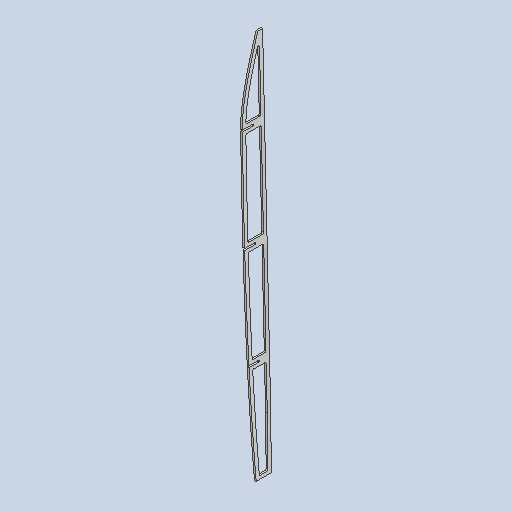
# Autodesk Inventor part: stringer_cowl
Saved by Autodesk Inventor 2022 (Build 260153000, 153)
## iProperties
Created: 2021-05-01
Part Number: stringer_cowl
Material: Generic
Document SubType Name: Modeling
Designer: kardo
Density: 1 g/cm^3
Appearance: Default
Mass: 8.25745 g
Surface Area: 121.112 cm^2
Volume: 8.25745 cm^3
Author: kardo
Autodesk Inventor part; units mm, degrees
ref_plane "YZ Plane" through (0, 0, 0) normal (1, 0, 0) x (0, 1, 0)
ref_plane "XZ Plane" through (0, 0, 0) normal (0, 1, 0) x (-1, 0, 0)
ref_plane "XY Plane" through (0, 0, 0) normal (0, 0, 1) x (1, 0, 0)
derived "frame_outline.ipt"
sketch "stringer_cowl" plane through (55, 0, 0) normal (1, 0, 0) x (0, 1, 0)
  line L0 (-363, 18.496) -> (-297.6664, 19.4083)
  line L1 (-37.9005, 25.6108) -> (-277.6703, 19.7906)
  line L2 (28.4595, 27.2216) -> (-37.9005, 25.6108)
  line L3 (94.8, 28.832) -> (28.4595, 27.2216)
  line L4 (-361, 19.324) -> (-297.6775, 20.2082)
  line L5 (-277.6897, 20.5903) -> (-37.9199, 26.4106)
  line L6 (-37.9199, 26.4106) -> (28.4401, 28.0214)
  line L7 (28.4401, 28.0214) -> (92.8, 29.5837)
  line L8 (-361, 19.324) -> (-361, 37.0229)
  line L9 (92.8, 35.2245) -> (92.8, 29.5837)
  line L10 (-363, 39.654) -> (-363, 18.496)
  spline S0 degree 3 poles (-297.6664, 19.4083) (-291.0004, 19.5014) (-284.3349, 19.6288) (-277.6703, 19.7906) knots 0 0 0 0 1 1 1 1
  spline S1 degree 3 poles (-297.6775, 20.2082) (-297.1223, 20.216) (-296.0117, 20.2319) (-294.6236, 20.2531) (-293.2355, 20.2752) (-292.125, 20.2936) (-290.7369, 20.3174) (-289.6264, 20.3372) (-288.2383, 20.3629) (-287.1279, 20.3841) (-285.7399, 20.4115) (-284.6295, 20.4342) (-283.2415, 20.4634) (-282.1311, 20.4875) (-280.7431, 20.5185) (-279.3552, 20.5504) (-278.2449, 20.5769) (-277.6897, 20.5903) knots 0 0 0 0 0.083333 0.166667 0.208333 0.291667 0.333333 0.416667 0.458333 0.541667 0.583333 0.666667 0.708333 0.791667 0.833333 0.916667 1 1 1 1
  line L11 (94.8, 37.536) -> (94.8, 28.832)
  spline S2 degree 2 poles (0, 55.974) (-217.9618, 52.7695) (-363, 39.654) knots 0 0 0 1 1 1
  spline S3 degree 4 poles (0, 55.974) (21.4177, 56.2889) (38.251, 53.3044) (69.464, 45.4203) (94.8, 37.536) knots 0 0 0 0 0 1 1 1 1 1
  spline S4 degree 3 poles (-361, 37.0229) (-344.9505, 38.4632) (-315.694, 40.8257) (-279.9192, 43.209) (-252.086, 44.8607) (-233.0296, 45.8939) (-208.5828, 47.1006) (-188.5245, 47.998) (-162.8256, 49.0348) (-141.7656, 49.7964) (-114.8147, 50.6634) (-92.7531, 51.289) (-64.5503, 51.9862) (-35.7216, 52.5983) (-11.991, 52.9974) (0.0412, 53.1743) knots 0 0 0 0 0.165663 0.28991 0.331326 0.414157 0.455573 0.538404 0.57982 0.662651 0.704067 0.786899 0.828314 0.911146 0.993977 0.993977 0.993977 0.993977
  spline S5 degree 3 poles (0.0412, 53.1743) (2.3587, 53.2084) (6.3001, 53.1906) (10.7199, 53.006) (14.0368, 52.795) (16.2548, 52.6178) (19.0489, 52.35) (21.306, 52.0987) (24.1648, 51.7379) (26.4854, 51.4121) (29.4354, 50.9585) (31.8372, 50.5588) (34.8963, 50.0138) (37.3902, 49.542) (40.5681, 48.9085) (43.1589, 48.3674) (46.4574, 47.6498) (49.1434, 47.0435) (52.5567, 46.2473) (55.3302, 45.5808) (58.8447, 44.7132) (61.6917, 43.9926) (65.2863, 43.0618) (68.1868, 42.2943) (71.8327, 41.31) (74.7608, 40.5039) (79.1539, 39.2715) (84.9974, 37.5914) (90.01, 36.0859) (92.8, 35.2245) knots 0 0 0 0 0.082372 0.144151 0.164743 0.205929 0.226522 0.267708 0.288301 0.329487 0.35008 0.391266 0.411859 0.453044 0.473637 0.514823 0.535416 0.576602 0.597195 0.638381 0.658974 0.70016 0.720753 0.761938 0.782531 0.823717 0.84431 0.906089 0.988461 0.988461 0.988461 0.988461
  point P0 (0, 0)
  point P1 (-242, 33.6806)
  point P2 (-121, 37.5562)
  point P3 (0, 40.4654)
  point P4 (94.8, 33.184)
  point P5 (-363, 28.288)
extrude "Extrusion1" add sketch "stringer_cowl" along normal blind 2 contours L8 S4 S5 L9 L7 L6 L5 S1 L4
sketch "Sketch2" plane through (55, -361, 19.324) normal (-1, 0, 0) x (0, 0, 1)
  line L0 (1.2663, 83.3103) -> (10.2597, 453.8) projected
  line L1 (1.2663, 83.3103) -> (10.2597, 453.8) projected
  line L2 (21.1414, 361) -> (21.1414, 363)
  line L3 (21.1414, 363) -> (38.8686, 363)
  line L4 (31.1344, 240) -> (18.2322, 240)
  line L5 (18.2322, 240) -> (18.2322, 242)
  line L6 (18.2322, 242) -> (31.1961, 242)
  line L7 (21.1414, 361) -> (38.8686, 361)
  line L8 (26.0756, 119) -> (14.3566, 119)
  line L9 (14.3566, 119) -> (14.3566, 121)
  line L10 (14.3566, 121) -> (26.1833, 121)
  line L11 (38.8686, 363) -> (38.8686, 361)
  spline S0 degree 3 poles (33.8503, 361.0412) (33.6734, 349.009) (33.2743, 325.2784) (32.6622, 296.4497) (31.965, 268.2469) (31.3394, 246.1853) (30.4724, 219.2344) (29.7108, 198.1744) (28.674, 172.4755) (27.7766, 152.4172) (26.5699, 127.9704) (25.5367, 108.914) (23.885, 81.0808) (21.5017, 45.306) (19.1392, 16.0495) (17.6989, 0) knots 0 0 0 0 0.083333 0.166667 0.208333 0.291667 0.333333 0.416667 0.458333 0.541667 0.583333 0.666667 0.708333 0.833333 1 1 1 1 projected
  point P0 (33.8686, 363)
  dimension "d4" = 2
  dimension "d5" = 2
  dimension "d6" = 2
  dimension "d18" = 5
  constraints: 20 end point, 6 horizontal, 4 vertical, 1 point on line, 7 other
  measures "d4" distance between parallel lines of L7 L3
  measures "d5" distance between parallel lines of L4 L6
  measures "d6" distance between parallel lines of L8 L10
  measures "d18" distance from line of L11 point (33.869, 363)
extrude "Extrusion2" cut sketch "Sketch2" against normal through all
sketch "Sketch3" plane through (55, -361, 19.324) normal (-1, 0, 0) x (0, 0, 1)
  line L0 (21.1414, 361) -> (33.8497, 361) projected
  line L1 (21.1414, 363) -> (21.1414, 361) projected
  line L2 (33.8686, 363) -> (21.1414, 363) projected
  line L3 (10.2597, 453.8) -> (15.9005, 453.8) projected
  line L4 (1.2663, 83.3103) -> (10.2597, 453.8) projected
  arc A0 (1.2663, 83.3103) -> (0.8842, 63.3225) centre (1940.3442, 36.2407) ccw projected
  line L5 (0, 0) -> (0.8842, 63.3225) projected
  line L6 (17.6989, 0) -> (0, 0) projected
  spline S0 degree 3 poles (15.9005, 453.8) (16.7619, 451.01) (18.2674, 445.9974) (19.9475, 440.1539) (21.1799, 435.7608) (21.986, 432.8327) (22.9703, 429.1868) (23.7378, 426.2863) (24.6686, 422.6917) (25.3892, 419.8447) (26.2568, 416.3302) (26.9233, 413.5567) (27.7195, 410.1434) (28.3258, 407.4574) (29.0434, 404.1589) (29.5845, 401.5681) (30.218, 398.3902) (30.6898, 395.8963) (31.2348, 392.8372) (31.6345, 390.4354) (32.0881, 387.4854) (32.4139, 385.1648) (32.7747, 382.306) (33.026, 380.0489) (33.2937, 377.2548) (33.471, 375.0368) (33.682, 371.7199) (33.8404, 367.9275) (33.8749, 364.6355) (33.8686, 363) knots 0 0 0 0 0.085352 0.149367 0.170705 0.213381 0.234719 0.277396 0.298734 0.34141 0.362748 0.405424 0.426762 0.469439 0.490777 0.533453 0.554791 0.597467 0.618806 0.661482 0.68282 0.725496 0.746834 0.78951 0.810849 0.853525 0.874863 0.938877 1 1 1 1
  spline S1 degree 3 poles (26.0756, 119) (25.8084, 114.0608) (25.2713, 104.4426) (23.885, 81.0808) (21.5017, 45.306) (19.1392, 16.0495) (17.6989, 0) knots 0 0 0 0 0.114662 0.225329 0.557331 1 1 1 1
  line L7 (14.3566, 119) -> (26.0756, 119) projected
  line L8 (14.3566, 121) -> (14.3566, 119) projected
  line L9 (26.1833, 121) -> (14.3566, 121) projected
  spline S2 degree 3 poles (31.1344, 240) (30.9747, 234.8512) (30.4626, 218.9639) (29.7108, 198.1744) (28.674, 172.4755) (27.7766, 152.4172) (26.8537, 133.7192) (26.3946, 124.9388) (26.1833, 121) knots 0 0 0 0 0.122043 0.379349 0.508002 0.765308 0.893961 1 1 1 1
  line L10 (18.2322, 240) -> (31.1344, 240) projected
  line L11 (18.2322, 242) -> (18.2322, 240) projected
  line L12 (31.1961, 242) -> (18.2322, 242) projected
  spline S3 degree 3 poles (33.8497, 361) (33.673, 348.9819) (33.274, 325.2653) (32.6622, 296.4497) (31.975, 268.6493) (31.5181, 252.4878) (31.1961, 242) knots 0 0 0 0 0.288422 0.577173 0.721548 1 1 1 1
  line L13 (27.3159, 246) -> (9.2167, 246)
  line L14 (8.9739, 236) -> (27.0071, 236)
  line L15 (22.3905, 125) -> (6.2795, 125)
  line L16 (6.0368, 115) -> (21.8512, 115)
  line L17 (14.0392, 4) -> (4.0562, 4)
  line L18 (4.0562, 4) -> (4.8838, 63.2666)
  arc A1 (5.2652, 83.2132) -> (4.8838, 63.2666) centre (1940.3442, 36.2407) ccw
  line L19 (5.2652, 83.2132) -> (14.0721, 446.0253)
  line L20 (29.8355, 367) -> (12.1539, 367)
  line L21 (11.9111, 357) -> (29.7895, 357)
  line L22 (31.1961, 242) -> (18.2322, 242) projected
  line L23 (18.2322, 240) -> (31.1344, 240) projected
  line L24 (26.1833, 121) -> (14.3566, 121) projected
  line L25 (14.3566, 119) -> (26.0756, 119) projected
  line L26 (33.8686, 363) -> (21.1414, 363) projected
  line L27 (21.1414, 361) -> (33.8497, 361) projected
  spline S4 degree 4 poles (27.0071, 236) (26.1281, 208.2394) (25.0852, 180.4841) (23.854, 152.7359) (22.3905, 125) knots 0 0 0 0 0 1 1 1 1 1
  spline S5 degree 4 poles (21.8513, 115) (20.3212, 87.2222) (18.5477, 59.458) (16.487, 31.712) (14.0392, 4) knots 0 0 0 0 0 1 1 1 1 1
  spline S6 degree 5 poles (14.0721, 446.0253) (15.6655, 440.6468) (17.2005, 435.251) (18.6856, 429.8412) (21.6907, 418.4511) (24.3963, 406.9856) (25.7125, 400.9574) (27.7211, 390.5917) (29.0755, 380.1243) (29.4979, 375.7586) (29.7444, 371.3809) (29.8355, 367) knots 0 0 0 0 0 0 0.347108 0.347108 0.347108 0.728865 0.728865 0.728865 1 1 1 1 1 1
  spline S7 degree 3 poles (29.7895, 357) (29.2273, 319.9948) (28.4285, 282.9928) (27.3158, 246) knots 0 0 0 0 1 1 1 1
  dimension "d20" = 4
  dimension "d21" = 4
  dimension "d19" = 4
  dimension "d22" = 4
  constraints: 18 end point, 13 parallel, 6 point on line, 2 point on circle, 1 centre point, 19 other
  measures "d19" distance between parallel lines of L4 L19
  measures "d22" distance between parallel lines of L12 L13
extrude "Extrusion3" cut sketch "Sketch3" against normal through all contours L13 L19 L21 S7 | L14 S4 L15 L19 | L16 S5 L17 L18 A1 L19 | L19 S6 L20
fillet "Fillet1" radius 1.3333 15 edges at (56, 6, 31.4779) (56, -115, 28.5407) (56, -236, 25.6035) (56, -357, 23.3802) (56, -357, 33.3632) (56, -236, 41.7145) (56, -115, 46.6399) (56, 6, 49.1595) (56, -246, 25.3608) (56, -125, 28.2979) (56, -4, 31.2351) (56, -246, 41.1753) (56, -125, 46.3311) (56, -4, 49.1135) (56, 85.0253, 33.3961)
equation "\"d1\" = bulkhead_thickness"
equation "\"d4\" = bulkhead_thickness"
equation "\"d5\" = bulkhead_thickness"
equation "\"d6\" = bulkhead_thickness"
equation "\"d20\" = inset"
equation "\"d21\" = inset"
equation "\"d19\" = inset"
equation "\"d22\" = inset"
equation "\"d17\" = 0.333333 * inset"
equation "\"bulkhead_thickness\" = 2"
equation "\"inset\" = 4"
body "Solid1"
